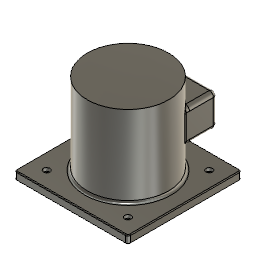
Robotic Arm (Autodesk Fusion 360 archive; units mm, degrees)
design "Base"
part number: 2026-08-18-15-37-16-751
Autodesk Fusion 360 part; units mm, degrees
note: some values were not read from the file. Chosen so that the rebuilt part matches the saved one: a direction; how an offset face is resized; which pieces of a blend or face edit are solid. Set by a fixed rule: which sketch regions a step uses.
sketch "Sketch1" plane through (0, 0, 0) normal (0, 0, 1) x (1, 0, 0)
  line L0 (70, 70) -> (-70, 70)
  line L1 (-70, 70) -> (-70, -70)
  line L2 (-70, -70) -> (70, -70)
  line L3 (70, -70) -> (70, 70)
  line L4 (70, 70) -> (-70, -70) construction
  line L5 (-70, 70) -> (70, -70) construction
  dimension "d1" = 140
  dimension "d2" = 140
  constraint horizontal L0
  constraint perpendicular L0 L1
  constraint parallel L0 L2
  constraint parallel L1 L3
  constraint coincident L4 origin
  constraint coincident L5 origin
  measures "d1" distance of L1.end L2.end
  measures "d2" distance of L0.end L1.end
extrude "Extrude1" add sketch "Sketch1" along normal blind 10
sketch "Sketch2" plane through (0, 0, 10) normal (0, 0, 1) x (-1, 0, 0)
  line L0 (-70, 70) -> (-70, -70)
  line L1 (-70, -70) -> (70, -70)
  line L2 (70, -70) -> (70, 70)
  line L3 (70, 70) -> (-70, 70)
  circle A0 centre (0, 0) radius 50
  dimension "d5" = 100
  constraint coincident A0.centre origin
  measures "d5" diameter of A0
extrude "Extrude2" add sketch "Sketch2" along normal blind 100 contours A0
sketch "Sketch3" plane through (0, 0, 0) normal (0, 1, 0) x (1, 0, 0)
  line L0 (-40, -80) -> (40, -80)
  line L1 (40, -80) -> (40, -40)
  line L2 (40, -40) -> (-40, -40)
  line L3 (-40, -40) -> (-40, -80)
  dimension "d8" = 80
  dimension "d9" = 40
  dimension "d10" = 40
  dimension "d11" = 40
  constraint horizontal L0
  constraint vertical L1
  constraint horizontal L2
  constraint vertical L3
  measures "d8" distance of L0.start L0.end
  measures "d9" distance of L0.start L2.end
  measures "d10" vertical distance of origin L2.end
  measures "d11" distance of origin L1
extrude "Extrude3" add sketch "Sketch3" along normal blind 70
sketch "Sketch4" plane through (0, 0, 110) normal (0, 0, 1) x (-1, 0, 0)
  circle A0 centre (0, 0) radius 50
  circle A1 centre (0, 0) radius 47.5
  dimension "d14" = 95
  constraint coincident A0.centre A1.centre
  measures "d14" diameter of A1
sketch "Sketch6" plane through (0, 0, 10) normal (0, 0, 1) x (-1, 0, 0)
  circle A0 centre (0, 0) radius 50
  line L0 (-70, 70) -> (-70, -70)
  line L1 (-70, -70) -> (70, -70)
  line L2 (70, -70) -> (70, 70)
  line L3 (70, 70) -> (-70, 70)
  point P0 (-50, 50)
  point P1 (50, 50)
  point P2 (50, -50)
  point P3 (-50, -50)
  dimension "d17" = 20
  dimension "d18" = 20
  dimension "d19" = 20
  dimension "d20" = 20
  dimension "d21" = 20
  dimension "d22" = 20
  dimension "d23" = 20
  dimension "d24" = 20
  measures "d17" distance of L0 P0
  measures "d18" distance of L3 P0
  measures "d19" distance of L3 P1
  measures "d20" distance of L2 P1
  measures "d21" distance of L2 P2
  measures "d22" distance of L1 P2
  measures "d23" distance of L1 P3
  measures "d24" distance of L0 P3
hole "Hole1" at (50, -50, 10) at (50, 50, 10) at (-50, 50, 10) at (-50, -50, 10) direction (0, 0, -1) diameter 4.5 depth 20 tip angle 118 counterbore diameter 8 counterbore depth 4
fillet "Fillet1" radius 3 4 edges at (-70, 70, 5) (70, 70, 5) (70, -70, 5) (-70, -70, 5)
fillet "Fillet2" radius 5 6 edges at (0, 70, 80) (0, 70, 40) (-40, 70, 60) (40, 70, 60) (-40, 30, 60) (40, 30, 60)
fillet "Fillet3" radius 3 1 edges at (46.6164, -18.0808, 10)
fillet "Fillet4" radius 1 16 edges at (-69.1213, -69.1213, 10) (0, -70, 10) (69.1213, -69.1213, 10) (70, 0, 10) (69.1213, 69.1213, 10) (0, 70, 10) (-69.1213, 69.1213, 10) (-70, 0, 10) (0, -70, 0) (69.1213, -69.1213, 0) (70, 0, 0) (69.1213, 69.1213, 0) (0, 70, 0) (-69.1213, 69.1213, 0) (-70, 0, 0) (-69.1213, -69.1213, 0)
fillet "Fillet5" radius 5 12 edges at (-40.2327, 30.1152, 80) (-40, 48.3114, 80) (-38.5355, 68.5355, 78.5355) (-40.2327, 30.1152, 40) (-40, 48.3114, 40) (-38.5355, 68.5355, 41.4645) (40.2327, 30.1152, 80) (40, 48.3114, 80) (38.5355, 68.5355, 78.5355) (40.2327, 30.1152, 40) (40, 48.3114, 40) (38.5355, 68.5355, 41.4645)

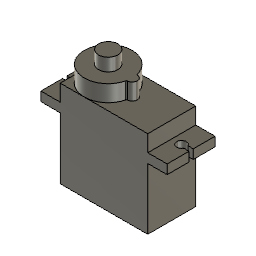
design "Servo"
part number: 2026-08-19-23-11-10-944
Autodesk Fusion 360 part; units mm, degrees
sketch "Sketch1" plane through (0, 0, 0) normal (0, 0, 1) x (1, 0, 0)
  line L0 (11.3, 6.2) -> (-11.3, 6.2)
  line L1 (-11.3, 6.2) -> (-11.3, -6.2)
  line L2 (-11.3, -6.2) -> (11.3, -6.2)
  line L3 (11.3, -6.2) -> (11.3, 6.2)
  line L4 (11.3, 6.2) -> (-11.3, -6.2) construction
  line L5 (-11.3, 6.2) -> (11.3, -6.2) construction
  dimension "d1" = 22.6
  dimension "d2" = 12.4
  constraint horizontal L0
  constraint perpendicular L0 L1
  constraint parallel L0 L2
  constraint parallel L1 L3
  constraint coincident L4 origin
  constraint coincident L5 origin
  measures "d1" distance of L1.end L2.end
  measures "d2" distance of L0.end L1.end
extrude "Extrude1" add sketch "Sketch1" along normal blind 22.5
sketch "Sketch2" plane through (0, 6.2, 0) normal (0, 1, 0) x (-1, 0, 0)
  line L0 (-11.3, 0) -> (11.3, 0)
  line L1 (11.3, 0) -> (11.3, 22.5)
  line L2 (11.3, 22.5) -> (-11.3, 22.5)
  line L3 (-11.3, 22.5) -> (-11.3, 0)
  line L4 (11.3, 18.25) -> (16.3, 18.25)
  line L5 (16.3, 18.25) -> (16.3, 15.85)
  line L6 (16.3, 15.85) -> (11.3, 15.85)
  line L7 (11.3, 15.85) -> (11.3, 18.25)
  line L8 (0, 22.5) -> (0, 0) construction
  line L9 (0, 22.5) -> (0, 0) construction
  line L10 (-11.3, 18.25) -> (-16.3, 18.25)
  line L11 (-16.3, 18.25) -> (-16.3, 15.85)
  line L12 (-16.3, 15.85) -> (-11.3, 15.85)
  dimension "d5" = 5
  dimension "d6" = 2.4
  dimension "d7" = 4.25
  constraint horizontal L4
  constraint vertical L5
  constraint horizontal L6
  constraint vertical L7
  constraint coincident L1 L4.start
  constraint midpoint L2 L8.start
  constraint coincident L8.end L9.end
  constraint symmetric L4.start L8 L10.start
  constraint symmetric L4.end L8 L10.end
  constraint symmetric L5.end L8 L11.end
  constraint symmetric L6.end L8 L12.end
  constraint symmetric L9.start L8 L8.start
  constraint symmetric L9.end L8 origin
  measures "d5" distance of L5.end L6.end
  measures "d6" distance of L4.end L5.end
  measures "d7" distance of L1.end L4
extrude "Extrude2" add sketch "Sketch2" against normal up to surface (12.4 mm away) contours L3 L10 L11 L12 | L1 L4 L5 L6 L7
sketch "Sketch3" plane through (0, 0, 18.25) normal (0, 0, 1) x (-1, 0, 0)
  line L0 (-11.3, 6.2) -> (-16.3, 6.2)
  line L1 (-16.3, 6.2) -> (-16.3, -6.2)
  line L2 (-16.3, -6.2) -> (-11.3, -6.2)
  line L3 (-11.3, -6.2) -> (-11.3, 6.2)
  line L4 (-16.3141, 0) -> (16.3141, 0) construction
  line L5 (0, -6) -> (0, 6) construction
  circle A0 centre (-13.8141, 0) radius 1.25
  line L6 (-16.3, 0.55) -> (-14.9366, 0.55)
  line L7 (-14.9366, 0.55) -> (-14.9366, -0.55)
  line L8 (-14.9366, -0.55) -> (-16.3, -0.55)
  line L9 (-16.3, -0.55) -> (-16.3, 0.55)
  dimension "d10" = 2.5
  dimension "d11" = 2.5
  dimension "d12" = 1.1
  constraint midpoint L4 origin
  constraint horizontal L4
  constraint midpoint L5 origin
  constraint perpendicular L4 L5
  constraint coincident L4 A0.centre
  constraint horizontal L6
  constraint vertical L7
  constraint horizontal L8
  constraint vertical L9
  constraint coincident L1 L6.start
  constraint coincident A0 L6.end
  constraint coincident A0 L7.end
  measures "d10" diameter of A0
  measures "d11" distance of L4.start A0.centre
  measures "d12" distance of L6.start L8.end
sketch "Sketch4" plane through (0, 0, 18.25) normal (0, 0, 1) x (-1, 0, 0)
extrude "Extrude3" cut sketch "Sketch3" against normal through all contours L1 A0 L6 L8 L9 | A0 L7 | A0 L7
sketch "Sketch5" plane through (0, 0, 18.25) normal (0, 0, 1) x (-1, 0, 0)
  line L0 (16.3, 6.2) -> (11.3, 6.2)
  line L1 (11.3, 6.2) -> (11.3, -6.2)
  line L2 (11.3, -6.2) -> (16.3, -6.2)
  line L3 (16.3, -6.2) -> (16.3, 6.2)
  line L4 (-16.3, 0) -> (16.3, 0) construction
  line L5 (0, 6.199) -> (0, -6.199) construction
  circle A0 centre (13.8, 0) radius 1.25
  line L6 (16.3, 0.55) -> (14.9225, 0.55)
  line L7 (14.9225, 0.55) -> (14.9225, -0.55)
  line L8 (14.9225, -0.55) -> (16.3, -0.55)
  line L9 (16.3, -0.55) -> (16.3, 0.55)
  dimension "d14" = 2.5
  dimension "d15" = 1.1
  dimension "d16" = 2.5
  constraint midpoint L4 origin
  constraint coincident L3 L4.end
  constraint perpendicular L3 L4
  constraint midpoint L5 origin
  constraint perpendicular L4 L5
  constraint coincident L4 A0.centre
  constraint horizontal L6
  constraint vertical L7
  constraint horizontal L8
  constraint vertical L9
  constraint coincident L3 L6.start
  constraint coincident A0 L6.end
  constraint coincident A0 L7.end
  measures "d14" diameter of A0
  measures "d15" distance of L6.start L8.end
  measures "d16" distance of L3 A0.centre
extrude "Extrude4" cut sketch "Sketch5" against normal through all contours L3 A0 L6 L8 L9 | A0 L7 | A0 L7
sketch "Sketch6" plane through (0, 0, 22.5) normal (0, 0, 1) x (-1, 0, 0)
  line L0 (-11.3, 6.2) -> (-11.3, -6.2)
  line L1 (-11.3, -6.2) -> (11.3, -6.2)
  line L2 (11.3, -6.2) -> (11.3, 6.2)
  line L3 (11.3, 6.2) -> (-11.3, 6.2)
  line L4 (11.3, -18.6) -> (11.3, 6.2) construction
  line L5 (-11.3, 18.6) -> (-11.3, -6.2) construction
  line L6 (33.9, 0) -> (-11.3, 0) construction
  circle A0 centre (5.1, 0) radius 6.2
  circle A1 centre (-1.1, 0) radius 1.3
  point P0 (11.3, -6.2)
  point P1 (-11.3, 6.2)
  point P2 (11.3, 0)
  dimension "d18" = 12.4
  dimension "d19" = 2.6
  constraint midpoint L4 P0
  constraint coincident P0 L1.end
  constraint coincident L2.end L3.start
  constraint midpoint L5 P1
  constraint coincident L0.start L3.end
  constraint coincident L0.end L1.start
  constraint midpoint L6 P2
  constraint coincident L2 P2
  constraint coincident L0 L6.end
  constraint perpendicular L0 L6
  constraint coincident L6 A0.centre
  constraint tangent L4 A0
  constraint coincident A0 A1.centre
  constraint coincident L6 A1.centre
  measures "d18" diameter of A0
  measures "d19" diameter of A1
extrude "Extrude5" add sketch "Sketch6" along normal blind 4.25 contours A0 A1 | A0 A1 | A0 A1
fillet "Fillet1" radius 0.25 2 edges at (0.9637, -1.2928, 24.625) (0.9637, 1.2928, 24.625)
sketch "Sketch7" plane through (0, 0, 26.75) normal (0, 0, 1) x (-1, 0, 0)
  arc A0 (-0.9186, -1.4888) -> (-0.9186, 1.4888) centre (5.1, 0) ccw
  arc A1 (-1.1514, 1.299) -> (-0.9186, 1.4888) centre (-1.1613, 1.5488) ccw
  arc A2 (-1.1514, 1.299) -> (-1.1514, -1.299) centre (-1.1, 0) ccw
  arc A3 (-0.9186, -1.4888) -> (-1.1514, -1.299) centre (-1.1613, -1.5488) ccw
  circle A4 centre (5.1, 0) radius 2.5
  dimension "d24" = 5
  constraint concentric A0 A4
  measures "d24" diameter of A4
extrude "Extrude6" add sketch "Sketch7" along normal blind 3.3 contours A4

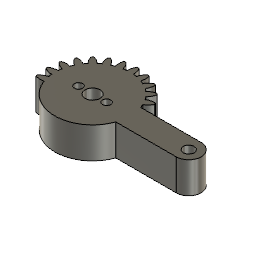
design "Gear"
part number: 2026-08-19-19-26-28-269
Autodesk Fusion 360 part; units mm, degrees
sketch "Sketch1" plane through (0, 0, 0) normal (0, 0, 1) x (1, 0, 0)
  circle A0 centre (0, 0) radius 12.09
  line L0 (0, 0) -> (30.75, 0)
  circle A1 centre (30.75, 0) radius 1.75
  circle A2 centre (0, 0) radius 1.75
  line L1 (0, -14.63) -> (0, 14.63) construction
  line L2 (0, 14.63) -> (-0.31, 14.63)
  line L3 (0, 14.63) -> (-0.31, 14.63)
  arc A3 (-0.31, 14.63) -> (-1.04, 12.0452) centre (3.9012, 12.0452) ccw
  arc A4 (1.04, 12.0452) -> (0.31, 14.63) centre (-3.9012, 12.0452) ccw
  line L4 (0.31, 14.63) -> (0, 14.63)
  arc A5 (-4.086, 14.0513) -> (-4.1221, 11.3656) centre (0.6508, 12.6445) ccw
  line L5 (-3.7865, 14.1315) -> (-4.086, 14.0513)
  line L6 (-3.4871, 14.2117) -> (-3.7865, 14.1315)
  arc A6 (-2.113, 11.9039) -> (-3.4871, 14.2117) centre (-6.8858, 10.625) ccw
  arc A7 (-7.5835, 12.515) -> (-6.9233, 9.9114) centre (-2.644, 12.382) ccw
  line L7 (-7.315, 12.67) -> (-7.5835, 12.515)
  line L8 (-7.0465, 12.825) -> (-7.315, 12.67)
  arc A8 (-5.1219, 10.9514) -> (-7.0465, 12.825) centre (-9.4011, 8.4808) ccw
  arc A9 (-10.5642, 10.1258) -> (-9.2526, 7.7818) centre (-5.7587, 11.2758) ccw
  line L9 (-10.345, 10.345) -> (-10.5642, 10.1258)
  line L10 (-10.1258, 10.5642) -> (-10.345, 10.345)
  arc A10 (-7.7818, 9.2526) -> (-10.1258, 10.5642) centre (-11.2758, 5.7587) ccw
  arc A11 (-12.825, 7.0465) -> (-10.9514, 5.1219) centre (-8.4808, 9.4011) ccw
  line L11 (-12.67, 7.315) -> (-12.825, 7.0465)
  line L12 (-12.515, 7.5835) -> (-12.67, 7.315)
  arc A12 (-9.9114, 6.9233) -> (-12.515, 7.5835) centre (-12.382, 2.644) ccw
  arc A13 (-14.2117, 3.4871) -> (-11.9039, 2.113) centre (-10.625, 6.8858) ccw
  line L13 (-14.1315, 3.7865) -> (-14.2117, 3.4871)
  line L14 (-14.0513, 4.086) -> (-14.1315, 3.7865)
  arc A14 (-11.3656, 4.1221) -> (-14.0513, 4.086) centre (-12.6445, -0.6508) ccw
  arc A15 (-14.63, -0.31) -> (-12.0452, -1.04) centre (-12.0452, 3.9012) ccw
  line L15 (-14.63, 0) -> (-14.63, -0.31)
  line L16 (-14.63, 0.31) -> (-14.63, 0)
  arc A16 (-12.0452, 1.04) -> (-14.63, 0.31) centre (-12.0452, -3.9012) ccw
  arc A17 (-14.0513, -4.086) -> (-11.3656, -4.1221) centre (-12.6445, 0.6508) ccw
  line L17 (-14.1315, -3.7865) -> (-14.0513, -4.086)
  line L18 (-14.2117, -3.4871) -> (-14.1315, -3.7865)
  arc A18 (-11.9039, -2.113) -> (-14.2117, -3.4871) centre (-10.625, -6.8858) ccw
  arc A19 (12.515, 7.5835) -> (9.9114, 6.9233) centre (12.382, 2.644) ccw
  line L19 (12.67, 7.315) -> (12.515, 7.5835)
  line L20 (12.825, 7.0465) -> (12.67, 7.315)
  arc A20 (10.9514, 5.1219) -> (12.825, 7.0465) centre (8.4808, 9.4011) ccw
  arc A21 (10.1258, 10.5642) -> (7.7818, 9.2526) centre (11.2758, 5.7587) ccw
  line L21 (10.345, 10.345) -> (10.1258, 10.5642)
  line L22 (10.5642, 10.1258) -> (10.345, 10.345)
  arc A22 (9.2526, 7.7818) -> (10.5642, 10.1258) centre (5.7587, 11.2758) ccw
  arc A23 (7.0465, 12.825) -> (5.1219, 10.9514) centre (9.4011, 8.4808) ccw
  line L23 (7.315, 12.67) -> (7.0465, 12.825)
  line L24 (7.5835, 12.515) -> (7.315, 12.67)
  arc A24 (6.9233, 9.9114) -> (7.5835, 12.515) centre (2.644, 12.382) ccw
  arc A25 (3.4871, 14.2117) -> (2.113, 11.9039) centre (6.8858, 10.625) ccw
  line L25 (3.7865, 14.1315) -> (3.4871, 14.2117)
  line L26 (4.086, 14.0513) -> (3.7865, 14.1315)
  arc A26 (4.1221, 11.3656) -> (4.086, 14.0513) centre (-0.6508, 12.6445) ccw
  circle A27 centre (30.75, 0) radius 4
  line L27 (30.75, 4) -> (11.4091, 4)
  line L28 (30.75, -4) -> (11.4091, -4)
  dimension "d1" = 24.18
  dimension "d2" = 30.75
  dimension "d3" = 3.5
  dimension "d4" = 3.5
  dimension "d5" = 29.26
  dimension "d6" = 0.31
  dimension "d9" = 360
  dimension "d10" = 8
  constraint coincident A0.centre L0.start
  constraint horizontal L0
  constraint coincident L0.end A1.centre
  constraint midpoint L1 A0.centre
  constraint perpendicular L0 L1
  constraint perpendicular L1 L2
  constraint perpendicular L1 L3
  constraint coincident A0 A3.end
  constraint symmetric L1 L2.end A4.end
  constraint symmetric L1 A3.end A4.start
  constraint symmetric L1 A3 A4
  constraint concentric A1 A27
  constraint coincident A27 L27.start
  constraint coincident A0 L27.end
  constraint tangent A27 L27
  constraint horizontal L27
  constraint coincident A27 L28.start
  constraint coincident A0 L28.end
  constraint tangent A27 L28
  constraint parallel L27 L28
  measures "d1" diameter of A0
  measures "d2" distance of A0.centre L0.end
  measures "d3" diameter of A1
  measures "d4" diameter of A2
  measures "d5" distance of L1.start L1.end
  measures "d6" distance of L1.end L2.end
  measures "d10" diameter of A27
extrude "Extrude1" add sketch "Sketch1" along normal blind 10
sketch "Sketch2" plane through (0, 0, 10) normal (0, 0, 1) x (-1, 0, 0)
  circle A0 centre (-30.75, 0) radius 1.75
  circle A1 centre (0, 0) radius 1.75
  line L0 (-30.75, -4) -> (-11.4091, -4)
  arc A2 (-11.4091, -4) -> (-10.9514, -5.1219) centre (0, 0) ccw
  arc A3 (-10.9514, -5.1219) -> (-12.825, -7.0465) centre (-8.4808, -9.4011) ccw
  line L1 (-12.825, -7.0465) -> (-12.515, -7.5835)
  arc A4 (-12.515, -7.5835) -> (-9.9114, -6.9233) centre (-12.382, -2.644) ccw
  arc A5 (-9.9114, -6.9233) -> (-9.2526, -7.7818) centre (0, 0) ccw
  arc A6 (-9.2526, -7.7818) -> (-10.5642, -10.1258) centre (-5.7587, -11.2758) ccw
  line L2 (-10.5642, -10.1258) -> (-10.1258, -10.5642)
  arc A7 (-10.1258, -10.5642) -> (-7.7818, -9.2526) centre (-11.2758, -5.7587) ccw
  arc A8 (-7.7818, -9.2526) -> (-6.9233, -9.9114) centre (0, 0) ccw
  arc A9 (-6.9233, -9.9114) -> (-7.5835, -12.515) centre (-2.644, -12.382) ccw
  line L3 (-7.5835, -12.515) -> (-7.0465, -12.825)
  arc A10 (-7.0465, -12.825) -> (-5.1219, -10.9514) centre (-9.4011, -8.4808) ccw
  arc A11 (-5.1219, -10.9514) -> (-4.1221, -11.3656) centre (0, 0) ccw
  arc A12 (-4.1221, -11.3656) -> (-4.086, -14.0513) centre (0.6508, -12.6445) ccw
  line L4 (-4.086, -14.0513) -> (-3.4871, -14.2117)
  arc A13 (-3.4871, -14.2117) -> (-2.113, -11.9039) centre (-6.8858, -10.625) ccw
  arc A14 (-2.113, -11.9039) -> (-1.04, -12.0452) centre (0, 0) ccw
  arc A15 (-1.04, -12.0452) -> (-0.31, -14.63) centre (3.9012, -12.0452) ccw
  line L5 (-0.31, -14.63) -> (0.31, -14.63)
  arc A16 (0.31, -14.63) -> (1.04, -12.0452) centre (-3.9012, -12.0452) ccw
  arc A17 (1.04, -12.0452) -> (2.113, -11.9039) centre (0, 0) ccw
  arc A18 (2.113, -11.9039) -> (3.4871, -14.2117) centre (6.8858, -10.625) ccw
  line L6 (3.4871, -14.2117) -> (4.086, -14.0513)
  arc A19 (4.086, -14.0513) -> (4.1221, -11.3656) centre (-0.6508, -12.6445) ccw
  arc A20 (4.1221, -11.3656) -> (5.1219, -10.9514) centre (0, 0) ccw
  arc A21 (5.1219, -10.9514) -> (7.0465, -12.825) centre (9.4011, -8.4808) ccw
  line L7 (7.0465, -12.825) -> (7.5835, -12.515)
  arc A22 (7.5835, -12.515) -> (6.9233, -9.9114) centre (2.644, -12.382) ccw
  arc A23 (6.9233, -9.9114) -> (7.7818, -9.2526) centre (0, 0) ccw
  arc A24 (7.7818, -9.2526) -> (10.1258, -10.5642) centre (11.2758, -5.7587) ccw
  line L8 (10.1258, -10.5642) -> (10.5642, -10.1258)
  arc A25 (10.5642, -10.1258) -> (9.2526, -7.7818) centre (5.7587, -11.2758) ccw
  arc A26 (9.2526, -7.7818) -> (9.9114, -6.9233) centre (0, 0) ccw
  arc A27 (9.9114, -6.9233) -> (12.515, -7.5835) centre (12.382, -2.644) ccw
  line L9 (12.515, -7.5835) -> (12.825, -7.0465)
  arc A28 (12.825, -7.0465) -> (10.9514, -5.1219) centre (8.4808, -9.4011) ccw
  arc A29 (10.9514, -5.1219) -> (11.3656, -4.1221) centre (0, 0) ccw
  arc A30 (11.3656, -4.1221) -> (14.0513, -4.086) centre (12.6445, 0.6508) ccw
  line L10 (14.0513, -4.086) -> (14.2117, -3.4871)
  arc A31 (14.2117, -3.4871) -> (11.9039, -2.113) centre (10.625, -6.8858) ccw
  arc A32 (11.9039, -2.113) -> (12.0452, -1.04) centre (0, 0) ccw
  arc A33 (12.0452, -1.04) -> (14.63, -0.31) centre (12.0452, 3.9012) ccw
  line L11 (14.63, -0.31) -> (14.63, 0.31)
  arc A34 (14.63, 0.31) -> (12.0452, 1.04) centre (12.0452, -3.9012) ccw
  arc A35 (12.0452, 1.04) -> (11.9039, 2.113) centre (0, 0) ccw
  arc A36 (11.9039, 2.113) -> (14.2117, 3.4871) centre (10.625, 6.8858) ccw
  line L12 (14.2117, 3.4871) -> (14.0513, 4.086)
  arc A37 (14.0513, 4.086) -> (11.3656, 4.1221) centre (12.6445, -0.6508) ccw
  arc A38 (11.3656, 4.1221) -> (-11.4091, 4) centre (0, 0) ccw
  line L13 (-11.4091, 4) -> (-30.75, 4)
  arc A39 (-30.75, 4) -> (-30.75, -4) centre (-30.75, 0) ccw
  line L14 (4.5, 0) -> (-4.5, 0) construction
  circle A40 centre (4.5, 0) radius 1.3
  circle A41 centre (-4.5, 0) radius 1.3
  dimension "d13" = 9
  dimension "d14" = 2.6
  dimension "d15" = 2.6
  constraint midpoint L14 A1.centre
  constraint coincident A1.centre A2.centre
  constraint horizontal L14
  constraint coincident L14.start A40.centre
  constraint coincident L14.end A41.centre
  measures "d13" distance of L14.start L14.end
  measures "d14" diameter of A40
  measures "d15" diameter of A41
sketch "Sketch3" plane through (0, 0, 10) normal (0, 0, 1) x (-1, 0, 0)
extrude "Extrude2" cut sketch "Sketch2" against normal blind 10 contours A40
extrude "Extrude3" cut sketch "Sketch2" against normal blind 10 contours A41
sketch "Sketch4" plane through (0, 0, 10) normal (0, 0, 1) x (-1, 0, 0)
  circle A0 centre (0, 0) radius 2.4
  dimension "d20" = 4.8
  constraint coincident A0.centre origin
  measures "d20" diameter of A0
extrude "Extrude4" cut sketch "Sketch4" against normal blind 10

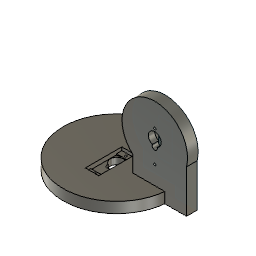
design "Base Link"
part number: 2026-08-19-17-00-12-411
Autodesk Fusion 360 part; units mm, degrees
sketch "Sketch1" plane through (0, 0, 0) normal (0, 0, 1) x (1, 0, 0)
  circle A0 centre (0, 0) radius 50
  dimension "d1" = 100
  constraint coincident A0.centre origin
  measures "d1" diameter of A0
extrude "Extrude1" add sketch "Sketch1" along normal blind 10
sketch "Sketch2" plane through (0, 0, 10) normal (0, 0, 1) x (-1, 0, 0)
  circle A0 centre (0, 0) radius 50
  line L0 (-6.25, -11) -> (6.25, -11)
  line L1 (6.25, -11) -> (6.25, 23)
  line L2 (6.25, 23) -> (-6.25, 23)
  line L3 (-6.25, 23) -> (-6.25, -11)
  line L4 (-6.25, -11) -> (6.25, 23) construction
  line L5 (6.25, -11) -> (-6.25, 23) construction
  line L6 (6.25, -6) -> (-6.25, -6)
  line L7 (6.25, 18) -> (-6.25, 18)
  point P0 (0, 6)
  point P1 (0, 6)
  dimension "d4" = 6
  dimension "d5" = 12.5
  dimension "d6" = 34
  dimension "d7" = 5
  dimension "d8" = 5
  constraint coincident A0.centre origin
  constraint horizontal L0
  constraint perpendicular L0 L1
  constraint parallel L0 L2
  constraint parallel L1 L3
  constraint coincident L4 P1
  constraint coincident L5 P1
  constraint coincident P1 P0
  constraint coincident L1 L6.start
  constraint coincident L3 L6.end
  constraint perpendicular L3 L6
  constraint coincident L1 L7.start
  constraint coincident L3 L7.end
  constraint perpendicular L3 L7
  measures "d4" distance of A0.centre P1
  measures "d5" distance of L1.end L2.end
  measures "d6" distance of L0.end L1.end
  measures "d7" distance of L0 L6
  measures "d8" distance of L2 L7
extrude "Extrude2" cut sketch "Sketch2" against normal blind 3 contours L0 L1 L3 L6 | L1 L3 L6 L7 | L1 L2 L3 L7
sketch "Sketch3" plane through (0, 0, 7) normal (0, 0, 1) x (-1, 0, 0)
  line L0 (-6.25, 23) -> (-6.25, -11)
  line L1 (-6.25, -11) -> (6.25, -11)
  line L2 (6.25, -11) -> (6.25, 23)
  line L3 (6.25, 23) -> (-6.25, 23)
  line L4 (6.25, -6) -> (-6.25, -6)
  line L5 (6.25, 18) -> (-6.25, 18)
  dimension "d11" = 5
  dimension "d12" = 5
  constraint coincident L2 L4.start
  constraint coincident L0 L4.end
  constraint perpendicular L0 L4
  constraint coincident L2 L5.start
  constraint coincident L0 L5.end
  constraint perpendicular L0 L5
  measures "d11" distance of L1 L4
  measures "d12" distance of L3 L5
extrude "Extrude3" cut sketch "Sketch3" against normal blind 1 contours L0 L2 L4 L5
sketch "Sketch4" plane through (0, 0, 6) normal (0, 0, 1) x (-1, 0, 0)
  line L0 (6.25, -6) -> (6.25, 18)
  line L1 (6.25, 18) -> (-6.25, 18)
  line L2 (-6.25, 18) -> (-6.25, -6)
  line L3 (-6.25, -6) -> (6.25, -6)
  circle A0 centre (0, 0) radius 6
  circle A1 centre (0, 6.5) radius 2.5
  dimension "d15" = 12
  dimension "d16" = 5
  dimension "d17" = 6.5
  constraint tangent L3 A0
  measures "d15" diameter of A0
  measures "d16" diameter of A1
  measures "d17" distance of A0.centre A1.centre
extrude "Extrude4" cut sketch "Sketch4" against normal blind 6 contours A0 A1 | A0 A1 | A0 A1
sketch "Sketch5" plane through (0, 0, 7) normal (0, 0, 1) x (-1, 0, 0)
  line L0 (-6.25, 18) -> (6.25, 18)
  line L1 (6.25, 18) -> (6.25, 23)
  line L2 (6.25, 23) -> (-6.25, 23)
  line L3 (-6.25, 23) -> (-6.25, 18)
  circle A0 centre (0, 20.5) radius 1.25
  dimension "d20" = 2.5
  dimension "d21" = 2.5
  measures "d20" diameter of A0
  measures "d21" distance of L2 A0.centre
sketch "Sketch6" plane through (0, 0, 7) normal (0, 0, 1) x (-1, 0, 0)
  line L0 (6.25, -6) -> (-6.25, -6)
  line L1 (-6.25, -6) -> (-6.25, -11)
  line L2 (-6.25, -11) -> (6.25, -11)
  line L3 (6.25, -11) -> (6.25, -6)
  circle A0 centre (0, -8.5) radius 1.25
  dimension "d22" = 2.5
  dimension "d23" = 2.5
  measures "d22" diameter of A0
  measures "d23" distance of L0 A0.centre
extrude "Extrude5" cut sketch "Sketch6" against normal through all contours A0
extrude "Extrude6" cut sketch "Sketch5" against normal through all contours A0
thread "Thread1" "ISO Metric profile 2.5 M2.5x0.45 M2.5x0.45 6H" major diameter 2.58 minor diameter 2.0755 pitch 0.45 angle 60 resizes the face on face at (-1.2438, -20.3755, 4.6667)
thread "Thread2" "ISO Metric profile 2.5 M2.5x0.45 M2.5x0.45 6H" major diameter 2.58 minor diameter 2.0755 pitch 0.45 angle 60 resizes the face on face at (-1.2438, 8.6245, 4.6667)
sketch "Sketch7" plane through (0, 0, 0) normal (0, 1, 0) x (1, 0, 0)
  line L0 (20, 0) -> (70, 0)
  line L1 (70, 0) -> (70, -40)
  arc A0 (20, -25) -> (70, -40) centre (40.4442, -47.6861) ccw
  line L2 (20, -25) -> (20, 0)
  dimension "d30" = 50
  dimension "d31" = 40
  dimension "d32" = 20
  constraint horizontal L0
  constraint perpendicular L0 L1
  constraint perpendicular L0 L2
  measures "d30" distance of L0.start L0.end
  measures "d31" distance of L0.end L1.end
  measures "d32" distance of origin L0.start
extrude "Extrude7" add sketch "Sketch7" along normal mid plane 10
sketch "Sketch8" plane through (0, 5, 0) normal (0, 1, 0) x (-1, 0, 0)
  line L0 (-49.7494, 10) -> (-20, 10)
  line L1 (-20, 10) -> (-20, 25)
  arc A0 (-20, 25) -> (-70, 40) centre (-40.4442, 47.6861) ccw
  line L2 (-70, 40) -> (-70, 0)
  line L3 (-70, 0) -> (-49.7494, 0)
  line L4 (-49.7494, 0) -> (-49.7494, 10)
  line L5 (-34.1942, 24.6861) -> (-46.6942, 24.6861)
  line L6 (-46.6942, 24.6861) -> (-46.6942, 58.6861)
  line L7 (-46.6942, 58.6861) -> (-34.1942, 58.6861)
  line L8 (-34.1942, 58.6861) -> (-34.1942, 24.6861)
  line L9 (-34.1942, 24.6861) -> (-46.6942, 58.6861) construction
  line L10 (-46.6942, 24.6861) -> (-34.1942, 58.6861) construction
  point P0 (-40.4442, 47.6861)
  point P1 (-40.4442, 41.6861)
  point P2 (-40.4442, 41.6861)
  dimension "d35" = 6
  dimension "d36" = 12.5
  dimension "d37" = 34
  constraint coincident P0 A0.centre
  constraint horizontal L5
  constraint perpendicular L5 L6
  constraint parallel L5 L7
  constraint parallel L6 L8
  constraint coincident L9 P2
  constraint coincident L10 P2
  constraint coincident P2 P1
  measures "d35" distance of P0 P2
  measures "d36" distance of L6.end L7.end
  measures "d37" distance of L5.end L6.end
extrude "Extrude8" cut sketch "Sketch8" against normal blind 3 contours L5 L6 L7 L8
sketch "Sketch9" plane through (0, 2, 0) normal (0, 1, 0) x (-1, 0, 0)
  line L0 (-34.1942, 58.6861) -> (-46.6942, 58.6861)
  line L1 (-46.6942, 58.6861) -> (-46.6942, 24.6861)
  line L2 (-46.6942, 24.6861) -> (-34.1942, 24.6861)
  line L3 (-34.1942, 24.6861) -> (-34.1942, 58.6861)
  line L4 (-46.6942, 53.6861) -> (-34.1942, 53.6861)
  line L5 (-46.6942, 29.6861) -> (-34.1942, 29.6861)
  dimension "d40" = 5
  dimension "d41" = 5
  constraint coincident L1 L4.start
  constraint coincident L3 L4.end
  constraint perpendicular L3 L4
  constraint coincident L1 L5.start
  constraint coincident L3 L5.end
  constraint perpendicular L3 L5
  measures "d40" distance of L0 L4
  measures "d41" distance of L2 L5
extrude "Extrude9" cut sketch "Sketch9" against normal blind 1 contours L1 L3 L4 L5
sketch "Sketch10" plane through (0, 1, 0) normal (0, 1, 0) x (-1, 0, 0)
  line L0 (-46.6942, 53.6861) -> (-46.6942, 29.6861)
  line L1 (-46.6942, 29.6861) -> (-34.1942, 29.6861)
  line L2 (-34.1942, 29.6861) -> (-34.1942, 53.6861)
  line L3 (-34.1942, 53.6861) -> (-46.6942, 53.6861)
  circle A0 centre (-40.4442, 47.6861) radius 6
  circle A1 centre (-40.4442, 41.1861) radius 2.5
  dimension "d44" = 12
  dimension "d45" = 5
  dimension "d46" = 6.5
  constraint tangent L3 A0
  measures "d44" diameter of A0
  measures "d45" diameter of A1
  measures "d46" distance of A0.centre A1.centre
extrude "Extrude10" cut sketch "Sketch10" against normal blind 6 contours A0 A1 | A0 A1 | A0 A1
sketch "Sketch11" plane through (0, 2, 0) normal (0, 1, 0) x (-1, 0, 0)
  line L0 (-34.1942, 29.6861) -> (-46.6942, 29.6861)
  line L1 (-46.6942, 29.6861) -> (-46.6942, 24.6861)
  line L2 (-46.6942, 24.6861) -> (-34.1942, 24.6861)
  line L3 (-34.1942, 24.6861) -> (-34.1942, 29.6861)
  circle A0 centre (-40.4442, 27.1861) radius 1.25
  dimension "d49" = 2.5
  dimension "d50" = 2.5
  measures "d49" diameter of A0
  measures "d50" distance of L2 A0.centre
sketch "Sketch12" plane through (0, 2, 0) normal (0, 1, 0) x (-1, 0, 0)
  line L0 (-46.6942, 53.6861) -> (-34.1942, 53.6861)
  line L1 (-34.1942, 53.6861) -> (-34.1942, 58.6861)
  line L2 (-34.1942, 58.6861) -> (-46.6942, 58.6861)
  line L3 (-46.6942, 58.6861) -> (-46.6942, 53.6861)
  circle A0 centre (-40.4442, 56.1861) radius 1.25
  dimension "d51" = 2.5
  dimension "d52" = 2.5
  measures "d51" diameter of A0
  measures "d52" distance of L0 A0.centre
extrude "Extrude11" cut sketch "Sketch12" against normal through all contours A0
extrude "Extrude12" cut sketch "Sketch11" against normal through all contours A0
thread "Thread3" "ISO Metric profile 2.5 M2.5x0.45 M2.5x0.45 6H" major diameter 2.58 minor diameter 2.0755 pitch 0.45 angle 60 resizes the face on face at (39.2004, -0.3333, 27.0616) on face at (41.596, -2.6667, 55.7005)
sketch "Sketch13" plane through (0, 5, 0) normal (0, 1, 0) x (-1, 0, 0)
  line L0 (-46.6942, 24.6861) -> (-46.6942, 58.6861)
  line L1 (-46.6942, 58.6861) -> (-34.1942, 58.6861)
  line L2 (-34.1942, 58.6861) -> (-34.1942, 24.6861)
  line L3 (-34.1942, 24.6861) -> (-46.6942, 24.6861)
  line L4 (-49.7494, 10) -> (-20, 10)
  line L5 (-20, 10) -> (-20, 25)
  arc A0 (-20, 25) -> (-70, 40) centre (-40.4442, 47.6861) ccw
  line L6 (-70, 40) -> (-70, 0)
  line L7 (-70, 0) -> (-49.7494, 0)
  line L8 (-49.7494, 0) -> (-49.7494, 10)

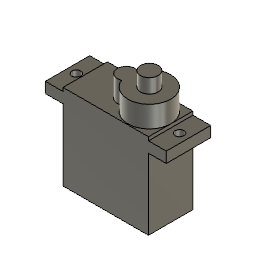
design "SG90"
part number: 2026-08-23-17-35-19-332
Autodesk Fusion 360 part; units mm, degrees
sketch "Sketch1" plane through (0, 0, 0) normal (0, 0, 1) x (1, 0, 0)
  line L0 (12, 6.25) -> (-12, 6.25)
  line L1 (-12, 6.25) -> (-12, -6.25)
  line L2 (-12, -6.25) -> (12, -6.25)
  line L3 (12, -6.25) -> (12, 6.25)
  line L4 (12, 6.25) -> (-12, -6.25) construction
  line L5 (-12, 6.25) -> (12, -6.25) construction
  line L6 (12, 6.25) -> (17, 6.25)
  line L7 (17, 6.25) -> (17, -6.25)
  line L8 (12, -6.25) -> (17, -6.25)
  line L9 (-12, 6.25) -> (-17, 6.25)
  line L10 (-17, 6.25) -> (-17, -6.25)
  line L11 (-17, -6.25) -> (-12, -6.25)
  dimension "d1" = 24
  dimension "d2" = 12.5
  dimension "d3" = 5
  dimension "d4" = 5
  constraint horizontal L0
  constraint perpendicular L0 L1
  constraint parallel L0 L2
  constraint parallel L1 L3
  constraint coincident L4 origin
  constraint coincident L5 origin
  constraint perpendicular L3 L6
  constraint perpendicular L2 L7
  constraint perpendicular L7 L8
  constraint perpendicular L1 L9
  constraint perpendicular L0 L10
  constraint perpendicular L1 L11
  measures "d1" distance of L1.end L2.end
  measures "d2" distance of L0.end L1.end
  measures "d3" distance of L0.start L6.end
  measures "d4" distance of L0.end L9.end
extrude "Extrude1" add sketch "Sketch1" along normal blind 24 contours L0 L1 L2 L3
sketch "Sketch2" plane through (0, -6.25, 0) normal (0, -1, 0) x (1, 0, 0)
  line L0 (-12, 0) -> (12, 0)
  line L1 (12, 0) -> (12, 24)
  line L2 (12, 24) -> (-12, 24)
  line L3 (-12, 24) -> (-12, 0)
  line L4 (12, 24) -> (12, 23)
  line L5 (12, 23) -> (17, 23)
  line L6 (17, 23) -> (17, 20)
  line L7 (17, 20) -> (12, 20)
  line L8 (-12, 24) -> (-12, 23)
  line L9 (-12, 23) -> (-17, 23)
  line L10 (-17, 23) -> (-17, 20)
  line L11 (-17, 20) -> (-12, 20)
  dimension "d7" = 1
  dimension "d8" = 5
  dimension "d9" = 3
  dimension "d10" = 1
  dimension "d11" = 5
  dimension "d12" = 3
  constraint coincident L1.end L2.start
  constraint perpendicular L2 L4
  constraint perpendicular L1 L5
  constraint perpendicular L5 L6
  constraint coincident L1 L7.end
  constraint perpendicular L1 L7
  constraint coincident L2.end L3.start
  constraint perpendicular L2 L8
  constraint perpendicular L3 L9
  constraint perpendicular L9 L10
  constraint coincident L3 L11.end
  constraint perpendicular L3 L11
  measures "d7" distance of L1.end L4.end
  measures "d8" distance of L4.end L5.end
  measures "d9" distance of L5.end L6.end
  measures "d10" distance of L2.end L8.end
  measures "d11" distance of L8.end L9.end
  measures "d12" distance of L9.end L10.end
extrude "Extrude2" add sketch "Sketch2" against normal up to surface (12.5 mm away) contours L3 L9 L10 L11 | L1 L5 L6 L7
sketch "Sketch3" plane through (0, 0, 24) normal (0, 0, 1) x (-1, 0, 0)
  line L0 (-12, 6.25) -> (-12, -6.25)
  line L1 (-12, -6.25) -> (12, -6.25)
  line L2 (12, -6.25) -> (12, 6.25)
  line L3 (12, 6.25) -> (-12, 6.25)
  circle A0 centre (-6, 0) radius 6
  circle A1 centre (0.5, 0) radius 2.5
  dimension "d15" = 12
  dimension "d16" = 5
  dimension "d17" = 6.5
  constraint tangent L0 A0
  measures "d15" diameter of A0
  measures "d16" diameter of A1
  measures "d17" distance of A0.centre A1.centre
extrude "Extrude3" add sketch "Sketch3" along normal blind 6 contours A0 A1 | A0 A1 | A0 A1
sketch "Sketch4" plane through (0, 0, 30) normal (0, 0, 1) x (-1, 0, 0)
  arc A0 (-0.4615, -2.3077) -> (-0.4615, 2.3077) centre (0.5, 0) ccw
  arc A1 (-0.4615, 2.3077) -> (-0.4615, -2.3077) centre (-6, 0) ccw
  circle A2 centre (-6, 0) radius 2.5
  dimension "d20" = 5
  constraint concentric A1 A2
  measures "d20" diameter of A2
extrude "Extrude4" add sketch "Sketch4" along normal blind 4 contours A2
sketch "Sketch5" plane through (0, 0, 23) normal (0, 0, 1) x (-1, 0, 0)
  line L0 (-17, -6.25) -> (-12, -6.25)
  line L1 (-12, -6.25) -> (-12, 6.25)
  line L2 (-12, 6.25) -> (-17, 6.25)
  line L3 (-17, 6.25) -> (-17, -6.25)
  circle A0 centre (-14.5, 0) radius 1.25
  dimension "d23" = 2.5
  dimension "d24" = 2.5
  measures "d23" diameter of A0
  measures "d24" distance of L3 A0.centre
sketch "Sketch6" plane through (0, 0, 23) normal (0, 0, 1) x (-1, 0, 0)
  line L0 (12, -6.25) -> (17, -6.25)
  line L1 (17, -6.25) -> (17, 6.25)
  line L2 (17, 6.25) -> (12, 6.25)
  line L3 (12, 6.25) -> (12, -6.25)
  circle A0 centre (14.5, 0) radius 1.25
  dimension "d25" = 2.5
  dimension "d26" = 2.5
  measures "d25" diameter of A0
  measures "d26" distance of L1 A0.centre
extrude "Extrude5" cut sketch "Sketch6" sketch "Sketch5" against normal blind 3 contours A0 of sketch 2 contours A0

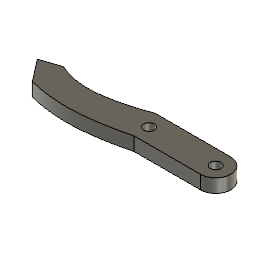
design "Gripper Holder 3.0"
part number: 2026-08-19-22-23-44-975
Autodesk Fusion 360 part; units mm, degrees
sketch "Sketch1" plane through (0, 0, 0) normal (0, 0, 1) x (1, 0, 0)
  line L0 (-11, 0) -> (11, 0) construction
  circle A0 centre (-11, 0) radius 1.75
  circle A1 centre (-11, 0) radius 5
  circle A2 centre (11, 0) radius 1.75
  circle A3 centre (11, 0) radius 5
  line L1 (-11, 5) -> (11, 5)
  line L2 (11, -5) -> (-11, -5)
  dimension "d1" = 22
  dimension "d2" = 3.5
  dimension "d3" = 10
  dimension "d4" = 3.5
  dimension "d5" = 10
  constraint midpoint L0 origin
  constraint horizontal L0
  constraint coincident L0.start A0.centre
  constraint concentric A0 A1
  constraint coincident L0.end A2.centre
  constraint concentric A2 A3
  constraint coincident A1 L1.start
  constraint coincident A3 L1.end
  constraint tangent A3 L1
  constraint coincident A3 L2.start
  constraint coincident A1 L2.end
  constraint tangent A1 L2
  measures "d1" distance of L0.start L0.end
  measures "d2" diameter of A0
  measures "d3" diameter of A1
  measures "d4" diameter of A2
  measures "d5" diameter of A3
extrude "Extrude1" add sketch "Sketch1" along normal blind 4.5
sketch "Sketch2" plane through (0, 0, 4.5) normal (0, 0, 1) x (-1, 0, 0)
  circle A0 centre (-11, 0) radius 1.75
  circle A1 centre (11, 0) radius 1.75
  arc A2 (11, -5) -> (11, 5) centre (11, 0) ccw
  line L0 (11, 5) -> (-11, 5)
  arc A3 (-11, 5) -> (-11, -5) centre (-11, 0) ccw
  line L1 (-11, -5) -> (11, -5)
  line L2 (11, 0) -> (11, -5) construction
  line L3 (0, 0) -> (0, 5) construction
  line L4 (11, 0) -> (11, 5) construction
  line L5 (0, 5) -> (11, 5)
  line L6 (13.99, -5) -> (11, -5)
  line L7 (13.99, -5) -> (11, -5)
  line L8 (13.99, -5) -> (11, -5)
  line L9 (0, 4.95) -> (0, 5.05)
  spline S0 degree 5 poles (43.3827, 6.2519) (42.8142, 6.3943) (41.6699, 6.6641) (39.9322, 7.0237) (37.572, 7.4115) (34.5449, 7.7335) (31.4348, 7.8797) (28.2359, 7.8379) (24.947, 7.6056) (21.5738, 7.1946) (18.1233, 6.6201) (15.3067, 6.0413) (13.1647, 5.5446) (11.7237, 5.1861) (11, 5) knots 0 0 0 0 0 0 0.1 0.2 0.3 0.4 0.5 0.6 0.7 0.8 0.9 1 1 1 1 1 1
  line L10 (49, -1) -> (43.3827, 6.2519)
  circle A4 centre (11, 0) radius 5
  line L11 (49, -1) -> (42.4735, -3.2067)
  spline S1 degree 5 poles (13.99, -5) (14.3125, -4.8777) (14.9644, -4.6352) (15.9628, -4.2778) (17.3358, -3.8142) (19.1224, -3.2581) (20.9787, -2.73) (22.901, -2.2385) (24.8802, -1.7975) (26.9002, -1.4266) (28.9415, -1.1487) (30.9832, -0.9869) (33.006, -0.962) (34.9943, -1.0892) (36.9392, -1.3746) (38.8366, -1.8183) (40.3155, -2.2977) (41.4029, -2.7258) (42.1182, -3.0414) (42.4735, -3.2067) knots 0 0 0 0 0 0 0.066667 0.133333 0.2 0.266667 0.333333 0.4 0.466667 0.533333 0.6 0.666667 0.733333 0.8 0.866667 0.933333 1 1 1 1 1 1
  point P0 (0, 5)
  point P1 (0, 5)
  point P2 (29.1574, 7.8223)
  point P3 (22.5528, -2.3387)
  point P4 (33, -1)
  dimension "d18" = 2.99
  dimension "d27" = 2.99
  dimension "d28" = 2.99
  constraint coincident A1.centre A2.centre
  constraint coincident A2.start L1.end
  constraint coincident L3.start origin
  constraint midpoint L0 P1
  constraint coincident A2.end L0.start
  constraint tangent A2 L6
  constraint coincident P1 P0
  constraint midpoint P1 L9
  constraint perpendicular L5 L9
  measures "d18" distance of A2.start L6.start
  measures "d27" distance of A2.start L6.start
  measures "d28" distance of A2.start L6.start
extrude "Extrude3" add sketch "Sketch2" against normal up to surface (4.5 mm away) contours A2 L6 L7 L8 S0 L10 A4 L11 S1
extrude "Extrude2" [suppressed]
